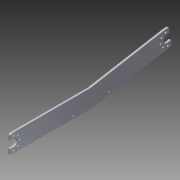
# Autodesk Inventor part: Arm_Link_1
Saved by Autodesk Inventor 2013 (Build 170138000, 138)
## iProperties
Created: 2014-05-15
Part Number: Arm_Link_1
Material: アルミニウム 6061
Document SubType Name: Modeling
Designer: andou
Density: 2.71 g/cm^3
Mass: 16.3631 g
Surface Area: 75.7922 cm^2
Volume: 6.03804 cm^3
Author: andou
Autodesk Inventor part; units mm, degrees
ref_plane "YZ Plane" through (0, 0, 0) normal (1, 0, 0) x (0, 1, 0)
ref_plane "XZ Plane" through (0, 0, 0) normal (0, 1, 0) x (-1, 0, 0)
ref_plane "XY Plane" through (0, 0, 0) normal (0, 0, 1) x (1, 0, 0)
sketch "スケッチ2" plane through (0, 0, 0) normal (1, 0, 0) x (0, 1, 0)
  line L0 (0, 0) -> (-84.4498, 0)
  line L1 (-84.4498, -20) -> (1.7498, -20)
  line L2 (0, 0) -> (83.1668, 14.6646)
  line L3 (86.6398, -5.0316) -> (1.7498, -20)
  arc A0 (87.251, 14.537) -> (83.1668, 14.6646) centre (84.9033, 4.8165) ccw
  arc A1 (86.6398, -5.0316) -> (90.434, -3.5148) centre (84.9033, 4.8165) ccw
  arc A2 (-88.4498, -19.1652) -> (-84.4498, -20) centre (-84.4498, -10) ccw
  arc A3 (-84.4498, 0) -> (-88.4498, -0.8348) centre (-84.4498, -10) ccw
  arc A4 (-84.4498, -14) -> (-84.4498, -6) centre (-84.4498, -10) ccw
  line L4 (-84.4498, -6) -> (-88.4498, -6)
  line L5 (-84.4498, -14) -> (-88.4498, -14)
  line L6 (-88.4498, -0.8348) -> (-88.4498, -6)
  line L7 (-88.4498, -14) -> (-88.4498, -19.1652)
  line L8 (87.251, 14.537) -> (88.1479, 9.4503)
  line L9 (89.5371, 1.5718) -> (90.434, -3.5148)
  line L10 (1.7498, -20) -> (0, 0)
  line L11 (88.1479, 9.4503) -> (89.5371, 1.5718)
  dimension "d21" = 20
  dimension "d22" = 10
  dimension "d23" = 170
  dimension "d27" = 10
  dimension "d31" = 8
  dimension "d33" = 4
  dimension "d35" = 4
  dimension "d36" = 170
  dimension "d139" = 20
  constraints: 24 end point, 10 point on circle, 8 perpendicular, 5 centre point, 4 equal length, 3 equal radius, 2 parallel, 2 tangent, 1 coincident, 1 collinear, 1 horizontal
  measures "d21" distance between parallel lines of L0 L1
  measures "d22" distance from line of L0 A2.centre
  measures "d23" angle of L0 L2
  measures "d27" radius of A3
  measures "d31" diameter of A4
  measures "d33" distance from line of L6 A2.centre
  measures "d35" distance from line of L8 L2.end
  measures "d36" distance of A2.centre A0.centre
  measures "d139" distance between parallel lines of L2 L3
extrude "押し出し1" add sketch "スケッチ2" along normal blind 2
sketch "スケッチ4" plane through (0, 0, 0) normal (-1, 0, 0) x (0, 0, 1)
  line L0 (-20, 1.7498) -> (-5.0316, 86.6398) projected
  line L1 (-20, -84.4498) -> (-20, 1.7498) projected
  circle A0 centre (-17, -18.5891) radius 1
  circle A1 centre (-13.5138, 21.2587) radius 1
  line L2 (-17, -18.5891) -> (-13.5138, 21.2587)
  line L3 (-20, 1.7498) -> (0, 0)
  dimension "d57" = 2
  dimension "d59" = 40
  dimension "d60" = 175
  dimension "d61" = 3
  dimension "d62" = 3
  constraints: 4 end point, 2 centre point, 1 equal radius
  measures "d57" diameter of A0
  measures "d59" distance of L2.start L2.end
  measures "d60" angle of L1 L2
  measures "d61" distance from line of L1 L2.start
  measures "d62" distance from line of L0 L2.end
hole "穴2" at (0, -18.5891, -17) at (0, 21.2587, -13.5138) direction (1, 0, 0) diameter 1.6 end through all
sketch "スケッチ6" plane through (2, 0, 0) normal (1, 0, 0) x (0, 0, -1)
  line L0 (20, 1.7498) -> (5.0316, 86.6398) projected
  arc A0 (5.0316, 86.6398) -> (3.5148, 90.434) centre (-4.8165, 84.9033) ccw projected
  line L1 (3.5148, 90.434) -> (-14.537, 87.251) projected
  arc A1 (-14.537, 87.251) -> (-14.6646, 83.1668) centre (-4.8165, 84.9033) ccw projected
  line L2 (-14.6646, 83.1668) -> (0, 0) projected
  line L3 (-9.3978, 53.2975) -> (-12.6117, 57.1277)
  line L4 (-14.537, 87.251) -> (-17.8212, 86.6719)
  line L5 (-17.8212, 86.6719) -> (-12.6117, 57.1277)
  line L6 (3.5148, 90.434) -> (6.799, 91.0131)
  line L7 (6.799, 91.0131) -> (12.0085, 61.4689)
  line L8 (12.0085, 61.4689) -> (10.2984, 56.7704)
  dimension "d75" = 150
  dimension "d76" = 150
  dimension "d77" = 2.5
  dimension "d78" = 2.5
  dimension "d79" = 30
  constraints: 12 end point, 3 parallel, 2 collinear, 2 point on line
  measures "d75" angle of L2 L3
  measures "d76" angle of L0 L8
  measures "d77" distance between parallel lines of L0 L7
  measures "d78" distance between parallel lines of L2 L5
  measures "d79" distance of L4.end L3.end
extrude "押し出し2" [suppressed]
sketch "スケッチ5" plane through (2, 0, 0) normal (1, 0, 0) x (0, 0, -1)
  line L0 (3.5148, 90.434) -> (-14.537, 87.251) projected
  circle A0 centre (-12.5213, 82.5293) radius 1.5
  circle A1 centre (3.2356, 85.3077) radius 1.5
  line L1 (5.0316, 86.6398) -> (20, 1.7498) projected
  line L2 (20, 1.7498) -> (20, -84.4498) projected
  arc A2 (19.1652, -88.4498) -> (20, -84.4498) centre (10, -84.4498) ccw projected
  line L3 (19.1652, -88.4498) -> (14, -88.4498) projected
  line L4 (14, -88.4498) -> (14, -84.4498) projected
  arc A3 (14, -84.4498) -> (6, -84.4498) centre (10, -84.4498) ccw projected
  line L5 (6, -84.4498) -> (6, -88.4498) projected
  line L6 (6, -88.4498) -> (0.8348, -88.4498) projected
  arc A4 (0, -84.4498) -> (0.8348, -88.4498) centre (10, -84.4498) ccw projected
  line L7 (0, -84.4498) -> (0, 0) projected
  line L8 (0, 0) -> (-14.6646, 83.1668) projected
  circle A5 centre (17, -18.5891) radius 0.8 projected
  circle A6 centre (13.5138, 21.2587) radius 0.8 projected
  arc A7 (-14.537, 87.251) -> (-14.6646, 83.1668) centre (-4.8165, 84.9033) ccw projected
  line L9 (-14.537, 87.251) -> (3.5148, 90.434) projected
  arc A8 (5.0316, 86.6398) -> (3.5148, 90.434) centre (-4.8165, 84.9033) ccw projected
  dimension "d70" = 5
  dimension "d71" = 5
  dimension "d72" = 3
  dimension "d114" = 16
  constraints: 2 centre point, 1 equal radius
  measures "d70" distance from line of L0 A0.centre
  measures "d71" distance from line of L0 A1.centre
  measures "d72" diameter of A1
  measures "d114" distance of A1.centre A0.centre
hole "穴3" [suppressed]
sketch "スケッチ7" plane through (2, 0, 0) normal (1, 0, 0) x (0, 0, -1)
  arc A0 (0, -84.4498) -> (0.8348, -88.4498) centre (10, -84.4498) ccw projected
  line L0 (0.8348, -88.4498) -> (6, -88.4498) projected
  circle A1 centre (3, -84.4498) radius 1
  dimension "d89" = 4
  dimension "d90" = 7
  dimension "d91" = 2
  constraints: 1 centre point
  measures "d89" distance from line of L0 A1.centre
  measures "d90" distance of A1.centre A0.centre
  measures "d91" diameter of A1
hole "穴4" at (2, -84.4498, -3) direction (-1, 0, 0) diameter 2 end through all
pattern_circular "円形状パターン3" count 5 over 180 about axis through (0, -84.4498, -10) along (-1, 0, 0) of "穴4"
sketch "スケッチ8" plane through (2, 0, 0) normal (1, 0, 0) x (0, 0, -1)
  line L0 (3.5148, 90.434) -> (-14.537, 87.251) projected
  line L1 (-17.8212, 86.6719) -> (-12.6117, 57.1277) projected
  circle A0 centre (-11.4794, 76.6205) radius 1.5
  circle A1 centre (4.2775, 79.3988) radius 1.5
  point P0 (6.799, 91.0131)
  dimension "d102" = 11
  dimension "d103" = 11
  dimension "d104" = 16
  dimension "d105" = 4.5
  dimension "d106" = 3
  constraints: 2 centre point, 1 equal radius
  measures "d102" distance from line of L0 A0.centre
  measures "d103" distance from line of L0 A1.centre
  measures "d104" distance of A1.centre A0.centre
  measures "d105" distance from line of L1 A0.centre
  measures "d106" diameter of A1
hole "穴5" [suppressed]
sketch "スケッチ11" plane through (2, 0, 0) normal (1, 0, 0) x (0, 0, -1)
  circle A0 centre (-11.4794, 76.6205) radius 1.75 projected
  circle A1 centre (4.2775, 79.3988) radius 1.75 projected
  line L0 (-17.8212, 86.6719) -> (-12.6117, 57.1277) projected
  circle A2 centre (-8.8747, 61.8483) radius 1.5
  circle A3 centre (6.8822, 64.6267) radius 1.5
  dimension "d124" = 3
  dimension "d126" = 16
  dimension "d127" = 15
  dimension "d128" = 4.5
  dimension "d130" = 15
  constraints: 2 centre point, 1 equal radius
  measures "d124" diameter of A2
  measures "d126" distance of A3.centre A2.centre
  measures "d127" distance of A0.centre A2.centre
  measures "d128" distance from line of L0 A2.centre
  measures "d130" distance of A1.centre A3.centre
hole "穴6" [suppressed]
sketch "スケッチ13" plane through (2, 0, 0) normal (1, 0, 0) x (0, 0, -1)
  line L0 (0, 0) -> (0, -84.4498) projected
  line L1 (20, -84.4498) -> (20, 1.7498) projected
  line L2 (20, 1.7498) -> (5.0316, 86.6398) projected
  line L3 (3.5148, 90.434) -> (-14.537, 87.251) projected
  line L4 (-14.6646, 83.1668) -> (0, 0) projected
  line L5 (-3.8662, 44.9615) -> (9.2538, 39.6592)
  line L6 (9.2538, 39.6592) -> (6.6491, 54.4313)
  line L7 (6.6491, 54.4313) -> (-3.8662, 44.9615)
  line L8 (-2.1297, 35.1134) -> (10.9903, 29.8111)
  line L9 (10.9903, 29.8111) -> (0.475, 20.3413)
  line L10 (0.475, 20.3413) -> (-2.1297, 35.1134)
  line L11 (2.7324, 7.5388) -> (13.2477, 17.0086)
  line L12 (13.2477, 17.0086) -> (15.8525, 2.2365)
  line L13 (15.8525, 2.2365) -> (2.7324, 7.5388)
  line L14 (4, -2.2635) -> (16, -9.7635)
  line L15 (4, -17.2635) -> (4, -2.2635)
  line L16 (16, -9.7635) -> (4, -17.2635)
  line L17 (4, -30.2635) -> (16, -22.7635)
  line L18 (16, -22.7635) -> (16, -37.7635)
  line L19 (16, -37.7635) -> (4, -30.2635)
  line L20 (4, -55.2635) -> (16, -47.7635)
  line L21 (16, -47.7635) -> (4, -40.2635)
  line L22 (4, -40.2635) -> (4, -55.2635)
  line L23 (4, -65.2635) -> (16, -57.7635)
  line L24 (16, -57.7635) -> (16, -72.7635)
  line L25 (16, -72.7635) -> (4, -65.2635)
  point P0 (10.2984, 56.7704)
  point P1 (6.799, 91.0131)
  point P2 (-17.8212, 86.6719)
  point P3 (-9.3978, 53.2975)
  dimension "d141" = 15
  dimension "d144" = 4
  dimension "d145" = 36
  dimension "d146" = 12
  dimension "d147" = 4
  dimension "d149" = 4
  dimension "d160" = 4
  dimension "d162" = 61
  dimension "d163" = 74
  dimension "d164" = 12
  dimension "d165" = 13
  dimension "d166" = 4
  dimension "d167" = 4
  dimension "d168" = 10
  dimension "d169" = 4
  dimension "d170" = 10
  constraints: 42 end point, 19 equal length, 8 parallel
  measures "d141" distance of L5.end L6.end
  measures "d144" distance between parallel lines of L2 L6
  measures "d145" distance from line of L3 L6.end
  measures "d146" distance from line of L5.start L6
  measures "d147" distance between parallel lines of L4 L10
  measures "d149" distance between parallel lines of L12 L2
  measures "d160" distance between parallel lines of L15 L0
  measures "d162" distance from line of L3 L8.end
  measures "d163" distance from line of L3 L11.end
  measures "d164" vertical distance of L12.end L14.end
  measures "d165" distance of L14.end L17.end
  measures "d166" distance between parallel lines of L1 L18
  measures "d167" distance between parallel lines of L0 L22
  measures "d168" distance of L18.end L20.end
  measures "d169" distance between parallel lines of L1 L24
  measures "d170" distance of L20.end L23.end
extrude "押し出し4" [suppressed]
fillet "フィレット1" [suppressed]
sketch "スケッチ14" plane through (2, 0, 0) normal (1, 0, 0) x (0, 0, -1)
  line L0 (3.5148, 90.434) -> (-14.537, 87.251) projected
  arc A0 (-14.537, 87.251) -> (-14.6646, 83.1668) centre (-4.8165, 84.9033) ccw projected
  arc A1 (-8.7557, 84.2087) -> (-0.8772, 85.5979) centre (-4.8165, 84.9033) ccw
  line L1 (-8.7557, 84.2087) -> (-9.4503, 88.1479)
  line L2 (-0.8772, 85.5979) -> (-1.5718, 89.5371)
  dimension "d174" = 8
  constraints: 4 end point, 2 perpendicular, 2 point on circle, 2 point on line, 2 tangent, 1 centre point, 1 coincident
  measures "d174" diameter of A1
extrude "押し出し5" cut sketch "スケッチ14" against normal blind 2
sketch "スケッチ15" plane through (2, 0, 0) normal (1, 0, 0) x (0, 0, -1)
  line L0 (-9.4503, 88.1479) -> (-14.537, 87.251) projected
  arc A0 (-14.537, 87.251) -> (-14.6646, 83.1668) centre (-4.8165, 84.9033) ccw projected
  circle A1 centre (-11.7101, 83.6878) radius 1
  dimension "d178" = 2
  dimension "d180" = 4
  dimension "d181" = 7
  constraints: 1 centre point
  measures "d178" diameter of A1
  measures "d180" distance from line of L0 A1.centre
  measures "d181" distance of A0.centre A1.centre
hole "穴7" at (2, 83.6878, 11.7101) direction (-1, 0, 0) diameter 2 end through all
pattern_circular "円形状パターン4" count 5 over 180 about axis through (2, 84.9033, 4.8165) along (1, 0, 0) of "穴7"
